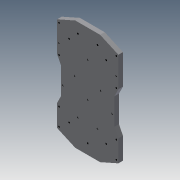
# Autodesk Inventor part: podvozek_komatex
Saved by Autodesk Inventor 2013 (Build 170138000, 138)
## iProperties
Created: 2012-09-03
Part Number: podvozek_komatex
Material: Generic
Document SubType Name: Modeling
Designer: idle-rug
Density: 1 g/cm^3
Author: idle-rug
Autodesk Inventor part; units mm, degrees
ref_plane "YZ Plane" through (0, 0, 0) normal (1, 0, 0) x (0, 1, 0)
ref_plane "XZ Plane" through (0, 0, 0) normal (0, 1, 0) x (-1, 0, 0)
ref_plane "XY Plane" through (0, 0, 0) normal (0, 0, 1) x (1, 0, 0)
sketch "Sketch1" plane through (0, 0, 0) normal (0, 1, 0) x (-1, 0, 0)
  circle A0 centre (24.1, 110.65) radius 0.25
  circle A1 centre (-70.5, 110.65) radius 0.25
  circle A2 centre (-45.6, 89.15) radius 0.25
  circle A3 centre (0, 67.65) radius 0.25
  circle A4 centre (70.5, 42.15) radius 0.25
  circle A5 centre (32.15, 17.15) radius 0.25
  circle A6 centre (60.5, -17.65) radius 0.25
  circle A7 centre (-60.5, -17.65) radius 0.25
  circle A8 centre (24.1, -67.65) radius 0.25
  circle A9 centre (-70.5, -67.65) radius 0.25
  circle A10 centre (-45.6, -89.15) radius 0.25
  circle A11 centre (0, -110.65) radius 0.25
  circle A12 centre (-70.5, -110.65) radius 0.25
  circle A13 centre (70.5, -110.65) radius 0.25
  circle A14 centre (45.6, -89.15) radius 0.25
  circle A15 centre (-24.1, -67.65) radius 0.25
  circle A16 centre (70.5, -67.65) radius 0.25
  circle A17 centre (0, -17.65) radius 0.25
  circle A18 centre (-32.15, 17.15) radius 0.25
  circle A19 centre (-70.5, 42.15) radius 0.25
  circle A20 centre (-70.5, 67.65) radius 0.25
  circle A21 centre (70.5, 67.65) radius 0.25
  circle A22 centre (45.6, 89.15) radius 0.25
  circle A23 centre (-24.1, 110.65) radius 0.25
  circle A24 centre (70.5, 110.65) radius 0.25
  line L0 (75.5, -115.65) -> (75.5, -62.65)
  line L1 (75.5, -62.65) -> (65.5, -42.65)
  line L2 (65.5, -42.65) -> (65.5, 22.15)
  line L3 (65.5, 22.15) -> (75.5, 42.15)
  line L4 (75.5, 42.15) -> (75.5, 115.65)
  line L5 (75.5, 115.65) -> (30.5, 135.65)
  line L6 (30.5, 135.65) -> (-30.5, 135.65)
  line L7 (-30.5, 135.65) -> (-75.5, 115.65)
  line L8 (-75.5, 115.65) -> (-75.5, 42.15)
  line L9 (-75.5, 42.15) -> (-65.5, 22.15)
  line L10 (-65.5, 22.15) -> (-65.5, -42.65)
  line L11 (-65.5, -42.65) -> (-75.5, -62.65)
  line L12 (-75.5, -62.65) -> (-75.5, -115.65)
  line L13 (-75.5, -115.65) -> (-30.5, -135.65)
  line L14 (-30.5, -135.65) -> (30.5, -135.65)
  line L15 (30.5, -135.65) -> (75.5, -115.65)
  circle A25 centre (0, -110.65) radius 2
  circle A26 centre (70.5, -110.65) radius 2
  circle A27 centre (-70.5, -110.65) radius 2
  circle A28 centre (45.6, -89.15) radius 2
  circle A29 centre (-45.6, -89.15) radius 2
  circle A30 centre (70.5, -67.65) radius 2
  circle A31 centre (24.1, -67.65) radius 2
  circle A32 centre (-24.1, -67.65) radius 2
  circle A33 centre (-70.5, -67.65) radius 2
  circle A34 centre (60.5, -17.65) radius 2
  circle A35 centre (0, -17.65) radius 2
  circle A36 centre (-32.15, 17.15) radius 2
  circle A37 centre (-60.5, -17.65) radius 2
  circle A38 centre (32.15, 17.15) radius 2
  circle A39 centre (70.5, 42.15) radius 2
  circle A40 centre (-70.5, 42.15) radius 2
  circle A41 centre (-70.5, 67.65) radius 2
  circle A42 centre (0, 67.65) radius 2
  circle A43 centre (70.5, 67.65) radius 2
  circle A44 centre (45.6, 89.15) radius 2
  circle A45 centre (-45.6, 89.15) radius 2
  circle A46 centre (-70.5, 110.65) radius 2
  circle A47 centre (-24.1, 110.65) radius 2
  circle A48 centre (24.1, 110.65) radius 2
  circle A49 centre (70.5, 110.65) radius 2
  point P0 (0, 0)
  point P1 (0, 0)
  dimension "d0" = 4
  dimension "d1" = 4
  dimension "d2" = 4
  dimension "d3" = 4
  dimension "d4" = 4
  dimension "d5" = 4
  dimension "d6" = 4
  dimension "d7" = 4
  dimension "d8" = 4
  dimension "d9" = 4
  dimension "d10" = 4
  dimension "d11" = 4
  dimension "d12" = 4
  dimension "d13" = 4
  dimension "d14" = 4
  dimension "d15" = 4
  dimension "d16" = 4
  dimension "d17" = 4
  dimension "d18" = 4
  dimension "d19" = 4
  dimension "d20" = 4
  dimension "d21" = 4
  dimension "d22" = 4
  dimension "d23" = 4
  dimension "d24" = 4
  constraints: 50 centre point, 32 end point, 25 coincident
  measures "d0" diameter of A25
  measures "d1" diameter of A26
  measures "d2" diameter of A27
  measures "d3" diameter of A28
  measures "d4" diameter of A29
  measures "d5" diameter of A30
  measures "d6" diameter of A31
  measures "d7" diameter of A32
  measures "d8" diameter of A33
  measures "d9" diameter of A34
  measures "d10" diameter of A35
  measures "d11" diameter of A36
  measures "d12" diameter of A37
  measures "d13" diameter of A38
  measures "d14" diameter of A39
  measures "d15" diameter of A40
  measures "d16" diameter of A41
  measures "d17" diameter of A42
  measures "d18" diameter of A43
  measures "d19" diameter of A44
  measures "d20" diameter of A45
  measures "d21" diameter of A46
  measures "d22" diameter of A47
  measures "d23" diameter of A48
  measures "d24" diameter of A49
extrude "Extrusion1" add sketch "Sketch1" along normal blind 2 contours L15 L14 L13 L12 L11 L10 L9 L8 L7 L6 L5 L4 L3 L2 L1 L0
sketch "Sketch2" plane through (0, 0, 0) normal (0, -1, 0) x (1, 0, 0)
  circle A0 centre (-70.5, 110.65) radius 2 projected
  circle A1 centre (-24.1, 110.65) radius 2 projected
  circle A2 centre (24.1, 110.65) radius 2 projected
  circle A3 centre (70.5, 110.65) radius 2 projected
  circle A4 centre (45.6, 89.15) radius 2 projected
  circle A5 centre (-45.6, 89.15) radius 2 projected
  circle A6 centre (-70.5, 67.65) radius 2 projected
  circle A7 centre (0, 67.65) radius 2 projected
  circle A8 centre (70.5, 67.65) radius 2 projected
  circle A9 centre (70.5, 42.15) radius 2 projected
  circle A10 centre (-70.5, 42.15) radius 2 projected
  circle A11 centre (-32.15, 17.15) radius 2 projected
  circle A12 centre (60.5, -17.65) radius 2 projected
  circle A13 centre (32.15, 17.15) radius 2 projected
  circle A14 centre (0, -17.65) radius 2 projected
  circle A15 centre (-60.5, -17.65) radius 2 projected
  circle A16 centre (70.5, -67.65) radius 2 projected
  circle A17 centre (24.1, -67.65) radius 2 projected
  circle A18 centre (-24.1, -67.65) radius 2 projected
  circle A19 centre (-70.5, -67.65) radius 2 projected
  circle A20 centre (45.6, -89.15) radius 2 projected
  circle A21 centre (-45.6, -89.15) radius 2 projected
  circle A22 centre (70.5, -110.65) radius 2 projected
  circle A23 centre (-70.5, -110.65) radius 2 projected
  circle A24 centre (0, -110.65) radius 2 projected
  line L0 (65.5, 22.15) -> (75.5, 42.15) projected
  line L1 (75.5, 42.15) -> (75.5, 115.65) projected
  line L2 (75.5, 115.65) -> (30.5, 135.65) projected
  line L3 (30.5, 135.65) -> (-30.5, 135.65) projected
  line L4 (-30.5, 135.65) -> (-75.5, 115.65) projected
  line L5 (-75.5, 115.65) -> (-75.5, 42.15) projected
  line L6 (-75.5, 42.15) -> (-65.5, 22.15) projected
  line L7 (-65.5, 22.15) -> (-65.5, -42.65) projected
  line L8 (-65.5, -42.65) -> (-75.5, -62.65) projected
  line L9 (-75.5, -62.65) -> (-75.5, -115.65) projected
  line L10 (-75.5, -115.65) -> (-30.5, -135.65) projected
  line L11 (-30.5, -135.65) -> (30.5, -135.65) projected
  line L12 (30.5, -135.65) -> (75.5, -115.65) projected
  line L13 (75.5, -115.65) -> (75.5, -62.65) projected
  line L14 (75.5, -62.65) -> (65.5, -42.65) projected
  line L15 (65.5, -42.65) -> (65.5, 22.15) projected
  point P0 (0, 0)
extrude "Extrusion2" add sketch "Sketch2" along normal blind 1.3
sketch "Sketch3" plane through (0, -1.3, 0) normal (0, -1, 0) x (1, 0, 0)
  circle A0 centre (0, -110.65) radius 2 projected
  circle A1 centre (-70.5, -110.65) radius 2 projected
  circle A2 centre (70.5, -110.65) radius 2 projected
  circle A3 centre (-45.6, -89.15) radius 2 projected
  circle A4 centre (45.6, -89.15) radius 2 projected
  circle A5 centre (-70.5, -67.65) radius 2 projected
  circle A6 centre (-24.1, -67.65) radius 2 projected
  circle A7 centre (24.1, -67.65) radius 2 projected
  circle A8 centre (70.5, -67.65) radius 2 projected
  circle A9 centre (-60.5, -17.65) radius 2 projected
  circle A10 centre (0, -17.65) radius 2 projected
  circle A11 centre (32.15, 17.15) radius 2 projected
  circle A12 centre (60.5, -17.65) radius 2 projected
  circle A13 centre (-32.15, 17.15) radius 2 projected
  circle A14 centre (-70.5, 42.15) radius 2 projected
  circle A15 centre (70.5, 42.15) radius 2 projected
  circle A16 centre (70.5, 67.65) radius 2 projected
  circle A17 centre (0, 67.65) radius 2 projected
  circle A18 centre (-70.5, 67.65) radius 2 projected
  circle A19 centre (-45.6, 89.15) radius 2 projected
  circle A20 centre (45.6, 89.15) radius 2 projected
  circle A21 centre (70.5, 110.65) radius 2 projected
  circle A22 centre (24.1, 110.65) radius 2 projected
  circle A23 centre (-24.1, 110.65) radius 2 projected
  circle A24 centre (-70.5, 110.65) radius 2 projected
  line L0 (65.5, 22.15) -> (75.5, 42.15) projected
  line L1 (75.5, 42.15) -> (75.5, 115.65) projected
  line L2 (75.5, 115.65) -> (30.5, 135.65) projected
  line L3 (30.5, 135.65) -> (-30.5, 135.65) projected
  line L4 (-30.5, 135.65) -> (-75.5, 115.65) projected
  line L5 (-75.5, 115.65) -> (-75.5, 42.15) projected
  line L6 (-75.5, 42.15) -> (-65.5, 22.15) projected
  line L7 (-65.5, 22.15) -> (-65.5, -42.65) projected
  line L8 (-65.5, -42.65) -> (-75.5, -62.65) projected
  line L9 (-75.5, -62.65) -> (-75.5, -115.65) projected
  line L10 (-75.5, -115.65) -> (-30.5, -135.65) projected
  line L11 (-30.5, -135.65) -> (30.5, -135.65) projected
  line L12 (30.5, -135.65) -> (75.5, -115.65) projected
  line L13 (75.5, -115.65) -> (75.5, -62.65) projected
  line L14 (75.5, -62.65) -> (65.5, -42.65) projected
  line L15 (65.5, -42.65) -> (65.5, 22.15) projected
  point P0 (0, 0)
extrude "Extrusion3" add sketch "Sketch3" along normal blind 8
sketch "Sketch4" plane through (0, 2, 0) normal (0, 1, 0) x (1, 0, 0)
  circle A0 centre (-32.15, -17.15) radius 2 projected
  circle A1 centre (60.5, 17.65) radius 2 projected
  circle A2 centre (32.15, -17.15) radius 2 projected
  circle A3 centre (0, 17.65) radius 2 projected
  circle A4 centre (-60.5, 17.65) radius 2 projected
  point P0 (0, 0)
extrude "Extrusion4" add sketch "Sketch4" against normal blind 10
sketch "Sketch5" plane through (0, 2, 0) normal (0, 1, 0) x (1, 0, 0)
  circle A0 centre (-70.5, -67.65) radius 2 projected
  circle A1 centre (0, -67.65) radius 2 projected
  circle A2 centre (70.5, -67.65) radius 2 projected
  circle A3 centre (24.1, 67.65) radius 2 projected
  circle A4 centre (-24.1, 67.65) radius 2 projected
  point P0 (0, 0)
extrude "Extrusion5" add sketch "Sketch5" against normal blind 10
body "Solid1"
